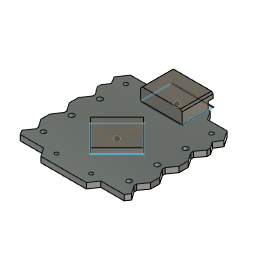
dfrobot_beetle (Autodesk Fusion 360 design; units mm, degrees)
Autodesk Fusion 360 part; units mm, degrees
sketch "Sketch1" plane through (0, 0, 0) normal (0, 0, 1) x (1, 0, 0)
  line L0 (0, 0) -> (120, 0)
  line L1 (120, 0) -> (120, 60)
  line L2 (120, 60) -> (0, 60)
  line L3 (0, 60) -> (0, 0)
  dimension "d1" = 120
  dimension "d2" = 60
  constraint horizontal L0
  constraint vertical L1
  constraint horizontal L2
  constraint vertical L3
  constraint coincident L0.start L3.end
  measures "d1" distance of L0.start L0.end
  measures "d2" distance of L0.start L2.end
extrude "Extrude1" add sketch "Sketch1" along normal blind 10 makes body 1
shell "Shell1" thickness 2 removed faces 1 at (40, 20, 10) on bodies 1
chamfer "Chamfer1" distance 3 angle 45 4 edges at (2, 58, 6) (118, 58, 6) (2, 2, 6) (118, 2, 6) on bodies 1
fillet "Fillet1" radius 3.5 8 edges at (2, 5, 6) (5, 2, 6) (115, 2, 6) (118, 5, 6) (118, 55, 6) (115, 58, 6) (5, 58, 6) (2, 55, 6) on bodies 1
sketch "Sketch1 (2)" plane through (0, 0, 0) normal (0, 0, 1) x (1, 0, 0) in component "beetle_board"
  line L0 (0, 11.4) -> (4.2, 11.4)
  line L1 (4.2, 11.4) -> (5.3, 9.8)
  line L2 (5.3, 9.8) -> (8.9, 9.8)
  line L3 (8.9, 9.8) -> (10.1, 8)
  line L4 (10.1, 8) -> (9.3, 6.7)
  line L5 (9.3, 6.7) -> (10.1, 5.5364)
  line L6 (10.1, 5.5364) -> (10.1, 4.9)
  line L7 (10.1, 4.9) -> (9.035, 3.481)
  line L8 (9.035, 3.481) -> (9.035, 3)
  line L9 (9.035, 3) -> (10.1, 1.4334)
  line L10 (10.1, 1.4334) -> (10.1, -0.2538)
  line L11 (10.1, -0.2538) -> (9.035, -1.7573)
  line L12 (9.035, -1.7573) -> (9.035, -2.25)
  line L13 (9.035, -2.25) -> (10.1, -3.8)
  line L14 (10.1, -3.8) -> (10.1, -5.5)
  line L15 (10.1, -5.5) -> (9.035, -6.9826)
  line L16 (9.035, -6.9826) -> (9.035, -7.4692)
  line L17 (9.035, -7.4692) -> (10.1, -8.9776)
  line L18 (10.1, -8.9776) -> (9.5675, -9.8011)
  line L19 (9.5675, -9.8011) -> (5.25, -9.8011)
  line L20 (5.25, -9.8011) -> (4.1787, -11.3908)
  line L21 (4.1787, -11.3908) -> (0, -11.3908)
  circle A0 centre (7.878, 7.9505) radius 0.3668
  circle A1 centre (7.878, 3.1799) radius 0.4655
  circle A2 centre (7.878, -2.0097) radius 0.4668
  circle A3 centre (7.878, -7.2117) radius 0.4322
  circle A4 centre (3.2, -9.5) radius 0.3291
  line L22 (0, 15) -> (0, -15) construction
  line L23 (-10.1, 1.4334) -> (-10.1, -0.2538)
  line L24 (-10.1, -3.8) -> (-10.1, -5.5)
  line L25 (-10.1, -0.2538) -> (-9.035, -1.7573)
  line L26 (-9.035, -6.9826) -> (-9.035, -7.4692)
  line L27 (-5.3, 9.8) -> (-8.9, 9.8)
  line L28 (-9.035, -1.7573) -> (-9.035, -2.25)
  circle A5 centre (-7.878, -7.2117) radius 0.4322
  line L29 (-9.035, -7.4692) -> (-10.1, -8.9776)
  line L30 (-9.035, -2.25) -> (-10.1, -3.8)
  line L31 (-10.1, -8.9776) -> (-9.5675, -9.8011)
  circle A6 centre (-7.878, 7.9505) radius 0.3668
  line L32 (-10.1, 8) -> (-9.3, 6.7)
  line L33 (0, 11.4) -> (-4.2, 11.4)
  line L34 (-10.1, 5.5364) -> (-10.1, 4.9)
  line L35 (-9.035, 3.481) -> (-9.035, 3)
  line L36 (-4.1787, -11.3908) -> (0, -11.3908)
  line L37 (-9.035, 3) -> (-10.1, 1.4334)
  line L38 (-4.2, 11.4) -> (-5.3, 9.8)
  line L39 (-10.1, 4.9) -> (-9.035, 3.481)
  line L40 (-8.9, 9.8) -> (-10.1, 8)
  line L41 (-9.5675, -9.8011) -> (-5.25, -9.8011)
  line L42 (-10.1, -5.5) -> (-9.035, -6.9826)
  circle A7 centre (-7.878, 3.1799) radius 0.4655
  line L43 (-9.3, 6.7) -> (-10.1, 5.5364)
  line L44 (-5.25, -9.8011) -> (-4.1787, -11.3908)
  circle A8 centre (-3.2, -9.5) radius 0.3291
  circle A9 centre (-7.878, -2.0097) radius 0.4668
  constraint horizontal L0
  constraint parallel L0 L2
  constraint parallel L1 L5
  constraint perpendicular L2 L6
  constraint parallel L6 L8
  constraint parallel L8 L10
  constraint parallel L10 L12
  constraint parallel L12 L14
  constraint parallel L14 L16
  constraint perpendicular L14 L19
  constraint parallel L19 L21
  constraint perpendicular L21 L22
  constraint symmetric L0.start L22 L33.start
  constraint symmetric L0.end L22 L33.end
  constraint symmetric L1.end L22 L27.start
  constraint symmetric L2.end L22 L27.end
  constraint symmetric L3.end L22 L32.start
  constraint symmetric L4.end L22 L32.end
  constraint symmetric L5.end L22 L34.start
  constraint symmetric L6.end L22 L34.end
  constraint symmetric L7.end L22 L35.start
  constraint symmetric L8.end L22 L35.end
  constraint symmetric L9.end L22 L23.start
  constraint symmetric L10.end L22 L23.end
  constraint symmetric L11.end L22 L25.end
  constraint symmetric L12.end L22 L28.end
  constraint symmetric L13.end L22 L24.start
  constraint symmetric L14.end L22 L24.end
  constraint symmetric L15.end L22 L26.start
  constraint symmetric L16.end L22 L26.end
  constraint symmetric L17.end L22 L29.end
  constraint symmetric L18.end L22 L31.end
  constraint symmetric L19.end L22 L41.end
  constraint symmetric L20.end L22 L36.start
  constraint symmetric L21.end L22 L36.end
  constraint symmetric A0 L22 A6
  constraint symmetric A1 L22 A7
  constraint symmetric A2 L22 A9
  constraint symmetric A3 L22 A5
  constraint symmetric A4 L22 A8
extrude "Extrude1'" add sketch "Sketch1 (2)" along normal blind 1.02 separate body makes body 2 in component "beetle_board"
sketch "Sketch2" plane through (0, 0, 1.02) normal (0, 0, 1) x (-1, 0, 0) in component "beetle_board"
  circle A0 centre (-7.878, -7.9505) radius 0.3668
  circle A1 centre (7.878, 2.0097) radius 0.4668
  circle A2 centre (3.2, 9.5) radius 0.3291
  circle A3 centre (7.878, -3.1799) radius 0.4655
  circle A4 centre (7.878, -7.9505) radius 0.3668
  circle A5 centre (7.878, 7.2117) radius 0.4322
  circle A6 centre (-3.2, 9.5) radius 0.3291
  circle A7 centre (-7.878, 7.2117) radius 0.4322
  circle A8 centre (-7.878, 2.0097) radius 0.4668
  circle A9 centre (-7.878, -3.1799) radius 0.4655
  line L0 (-4.2, -11.4) -> (4.2, -11.4)
  line L1 (4.2, -11.4) -> (5.3, -9.8)
  line L2 (5.3, -9.8) -> (8.9, -9.8)
  line L3 (8.9, -9.8) -> (10.1, -8)
  line L4 (10.1, -8) -> (9.3, -6.7)
  line L5 (9.3, -6.7) -> (10.1, -5.5364)
  line L6 (10.1, -5.5364) -> (10.1, -4.9)
  line L7 (10.1, -4.9) -> (9.035, -3.481)
  line L8 (9.035, -3.481) -> (9.035, -3)
  line L9 (9.035, -3) -> (10.1, -1.4334)
  line L10 (10.1, -1.4334) -> (10.1, 0.2538)
  line L11 (10.1, 0.2538) -> (9.035, 1.7573)
  line L12 (9.035, 1.7573) -> (9.035, 2.25)
  line L13 (9.035, 2.25) -> (10.1, 3.8)
  line L14 (10.1, 3.8) -> (10.1, 5.5)
  line L15 (10.1, 5.5) -> (9.035, 6.9826)
  line L16 (9.035, 6.9826) -> (9.035, 7.4692)
  line L17 (9.035, 7.4692) -> (10.1, 8.9776)
  line L18 (10.1, 8.9776) -> (9.5675, 9.8011)
  line L19 (9.5675, 9.8011) -> (5.25, 9.8011)
  line L20 (5.25, 9.8011) -> (4.1787, 11.3908)
  line L21 (4.1787, 11.3908) -> (-4.1787, 11.3908)
  line L22 (-4.1787, 11.3908) -> (-5.25, 9.8011)
  line L23 (-5.25, 9.8011) -> (-9.5675, 9.8011)
  line L24 (-9.5675, 9.8011) -> (-10.1, 8.9776)
  line L25 (-10.1, 8.9776) -> (-9.035, 7.4692)
  line L26 (-9.035, 7.4692) -> (-9.035, 6.9826)
  line L27 (-9.035, 6.9826) -> (-10.1, 5.5)
  line L28 (-10.1, 5.5) -> (-10.1, 3.8)
  line L29 (-10.1, 3.8) -> (-9.035, 2.25)
  line L30 (-9.035, 2.25) -> (-9.035, 1.7573)
  line L31 (-9.035, 1.7573) -> (-10.1, 0.2538)
  line L32 (-10.1, 0.2538) -> (-10.1, -1.4334)
  line L33 (-10.1, -1.4334) -> (-9.035, -3)
  line L34 (-9.035, -3) -> (-9.035, -3.481)
  line L35 (-9.035, -3.481) -> (-10.1, -4.9)
  line L36 (-10.1, -4.9) -> (-10.1, -5.5364)
  line L37 (-10.1, -5.5364) -> (-9.3, -6.7)
  line L38 (-9.3, -6.7) -> (-10.1, -8)
  line L39 (-10.1, -8) -> (-8.9, -9.8)
  line L40 (-8.9, -9.8) -> (-5.3, -9.8)
  line L41 (-5.3, -9.8) -> (-4.2, -11.4)
  line L42 (-3.815, -6.6) -> (3.815, -6.6)
  line L43 (3.815, -6.6) -> (3.815, -12.3)
  line L44 (3.815, -12.3) -> (-3.815, -12.3)
  line L45 (-3.815, -12.3) -> (-3.815, -6.6)
  line L46 (-3.815, -6.6) -> (3.815, -12.3) construction
  line L47 (3.815, -6.6) -> (-3.815, -12.3) construction
  line L48 (-4.879, 1.5692) -> (0, 6.4482)
  line L49 (0, 6.4482) -> (4.879, 1.5692)
  line L50 (4.879, 1.5692) -> (0, -3.3099)
  line L51 (0, -3.3099) -> (-4.879, 1.5692)
  line L52 (-4.879, 1.5692) -> (4.879, 1.5692) construction
  line L53 (0, 6.4482) -> (0, -3.3099) construction
  point P0 (0, -9.45)
  point P1 (0, 1.5692)
  dimension "d80" = 7.63
  dimension "d81" = 5.7
  dimension "d82" = 0.9
  dimension "d85" = 6.9
  dimension "d86" = 6.9
  constraint horizontal L42
  constraint perpendicular L42 L43
  constraint parallel L42 L44
  constraint parallel L43 L45
  constraint coincident L46 P0
  constraint coincident L47 P0
  constraint perpendicular L48 L49
  constraint parallel L48 L50
  constraint parallel L49 L51
  constraint coincident L52 P1
  constraint coincident L53 P1
  measures "d80" distance of L43.end L44.end
  measures "d81" distance of L42.end L43.end
  measures "d82" distance of L0 L44
  measures "d85" distance of L49.end L50.end
  measures "d86" distance of L48.end L49.end
extrude "Extrude2" add sketch "Sketch2" along normal blind 1 contours L48 L49 L50 L51 bodies 2 in component "beetle_board"
extrude "Extrude3" add sketch "Sketch2" along normal blind 2.4 contours L0 L42 L43 L45 | L0 L43 L44 L45 bodies 2 in component "beetle_board"
chamfer "Chamfer1'" distance 1.4 angle 45 2 edges at (3.815, 11.85, 1.02) (-3.815, 11.85, 1.02) on bodies 2 in component "beetle_board"
chamfer "Chamfer2" distance 0.3 angle 45 2 edges at (3.815, 9.45, 3.42) (-3.815, 9.45, 3.42) on bodies 2 in component "beetle_board"
component "beetle_board" placed x (1, 0, 0) y (0, 1, 0) z (0, 0, 1) at (0, 0, 0)
